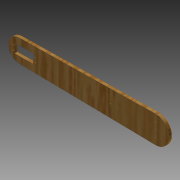
# Autodesk Inventor part: segment1
Saved by Autodesk Inventor 2013 (Build 170138000, 138)
## iProperties
Created: 2014-10-09
Part Number: segment1
Material: Plywood, Finish
Document SubType Name: Modeling
Designer: Masta
Density: 0.552 g/cm^3
Mass: 45.3224 g
Surface Area: 331.971 cm^2
Volume: 82.1058 cm^3
Author: Masta
Autodesk Inventor part; units mm, degrees
ref_plane "YZ Plane" through (0, 0, 0) normal (1, 0, 0) x (0, 1, 0)
ref_plane "XZ Plane" through (0, 0, 0) normal (0, 1, 0) x (-1, 0, 0)
ref_plane "XY Plane" through (0, 0, 0) normal (0, 0, 1) x (1, 0, 0)
sketch "Sketch1" plane through (0, 0, 0) normal (0, 1, 0) x (-1, 0, 0)
  line L0 (0, 0) -> (100, 0) construction
  line L1 (0, 0) -> (0, 15) construction
  line L2 (0, 0) -> (0, -15) construction
  arc A0 (0.545, 29.995) -> (0.545, -29.995) centre (0, 0) ccw
  line L3 (100, 0) -> (300, 0) construction
  line L4 (270, -10) -> (310.5, -10)
  line L5 (310.5, -10) -> (310.5, 10)
  line L6 (310.5, 10) -> (270, 10)
  line L7 (270, 10) -> (270, -10)
  line L8 (270, -10) -> (310.5, 10) construction
  line L9 (310.5, -10) -> (270, 10) construction
  line L10 (266, 5) -> (314.5, 5) construction
  line L11 (314.5, 5) -> (314.5, -5) construction
  line L12 (314.5, -5) -> (266, -5) construction
  line L13 (266, -5) -> (266, 5) construction
  line L14 (266, 5) -> (314.5, -5) construction
  line L15 (314.5, 5) -> (266, -5) construction
  arc A1 (0.545, 29.995) -> (300.3792, 24.9971) centre (1817.125, 100013.4939) ccw
  arc A2 (300.3792, -24.9971) -> (0.545, -29.995) centre (1817.125, -100013.4939) ccw
  arc A3 (300.3792, -24.9971) -> (300.3792, 24.9971) centre (300, 0) ccw
  point P0 (290.25, 0)
  dimension "d0" = 100
  dimension "d1" = 15
  dimension "d2" = 60
  dimension "d3" = 300
  dimension "d4" = 40.5
  dimension "d5" = 10.5
  dimension "d6" = 20
  dimension "d8" = 48.5
  dimension "d9" = 10
  dimension "d10" = 100000
  dimension "d11" = 25
  constraints: 32 end point, 10 coincident, 8 point on circle, 5 equal length, 4 centre point, 4 midpoint, 4 perpendicular, 3 horizontal, 3 symmetric about line, 2 tangent, 1 collinear, 1 point on line, 1 other
  measures "d0" distance of L0.start L0.end
  measures "d1" distance of L1.start L1.end
  measures "d2" diameter of A0
  measures "d3" distance of L1.start L3.end
  measures "d4" distance of L5.end L6.end
  measures "d5" distance from line of L5 L3.end
  measures "d6" distance of L4.end L5.end
  measures "d8" distance of L11.end L12.end
  measures "d9" distance of L10.end L11.end
  measures "d10" radius of A1
  measures "d11" radius of A3
extrude "Extrusion1" add sketch "Sketch1" along normal blind 6
hole "Hole1" at (0, 0, 0) at (-100, 0, 0) at (0, 0, 15) at (0, 0, -15) at (-266, 0, 5) at (-266, 0, -5) at (-314.5, 0, -5) at (-314.5, 0, 5) direction (0, 1, 0) diameter 3 end through all
body "Solid1"
